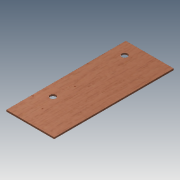
# Autodesk Inventor part: gabarito-contraponto
Saved by Autodesk Inventor 2017 (Build 210142000, 142)
## iProperties
Created: 2018-08-18
Part Number: gabarito-contraponto
Material: Wood (Oak)
Document SubType Name: Sheet Metal
Designer: Luiz Gustavo
Density: 0.76 g/cm^3
Sheet Metal Rule: Default_mm
Appearance: White Oak - Natural Medium Gloss
Author: Luiz Gustavo
Autodesk Inventor part; units mm, degrees
ref_plane "YZ Plane" through (0, 0, 0) normal (1, 0, 0) x (0, 1, 0)
ref_plane "XZ Plane" through (0, 0, 0) normal (0, 1, 0) x (-1, 0, 0)
ref_plane "XY Plane" through (0, 0, 0) normal (0, 0, 1) x (1, 0, 0)
sketch "Sketch1" plane through (0, 0, 0) normal (0, 0, 1) x (1, 0, 0)
  line L0 (-7.6357, 22.9943) -> (-8.4175, 23.9734) construction
  arc A0 (-7.6357, 22.9943) -> (-7.6357, 20.0058) centre (-4.4375, 21.5001) ccw construction
  line L1 (-8.4175, 19.0267) -> (-7.6357, 20.0058) construction
  arc A1 (-8.4175, 19.0267) -> (-6.9109, 17.5201) centre (-7.5798, 18.3578) ccw construction
  line L2 (-5.9318, 18.3019) -> (-6.9109, 17.5201) construction
  arc A2 (-5.9318, 18.3019) -> (-2.9433, 18.3019) centre (-4.4375, 21.5001) ccw construction
  line L3 (-1.9642, 17.5201) -> (-2.9433, 18.3019) construction
  arc A3 (-1.9642, 17.5201) -> (-0.4576, 19.0267) centre (-1.2953, 18.3578) ccw construction
  line L4 (-1.2394, 20.0058) -> (-0.4576, 19.0267) construction
  arc A4 (-1.2394, 20.0058) -> (-1.2394, 22.9943) centre (-4.4375, 21.5001) ccw construction
  line L5 (-0.4576, 23.9734) -> (-1.2394, 22.9943) construction
  arc A5 (-0.4576, 23.9734) -> (-1.9642, 25.48) centre (-1.2953, 24.6423) ccw construction
  line L6 (-2.9433, 24.6982) -> (-1.9642, 25.48) construction
  arc A6 (-2.9433, 24.6982) -> (-5.9318, 24.6982) centre (-4.4375, 21.5001) ccw construction
  line L7 (-6.9109, 25.48) -> (-5.9318, 24.6982) construction
  arc A7 (-6.9109, 25.48) -> (-8.4175, 23.9734) centre (-7.5798, 24.6423) ccw construction
  line L8 (-18.1375, 31.381) -> (-18.1375, 34.2) construction
  arc A8 (-18.1375, 31.381) -> (-17.7565, 31) centre (-17.7565, 31.381) ccw construction
  line L9 (-14.3175, 31) -> (-17.7565, 31) construction
  arc A9 (-14.3175, 31) -> (-13.9375, 31.38) centre (-14.3175, 31.38) ccw construction
  line L10 (-13.9375, 34.819) -> (-13.9375, 31.38) construction
  arc A10 (-13.9375, 34.819) -> (-14.3185, 35.2) centre (-14.3185, 34.819) ccw construction
  line L11 (-17.1375, 35.2) -> (-14.3185, 35.2) construction
  arc A11 (-17.1375, 35.2) -> (-18.1375, 34.2) centre (-17.1375, 34.2) ccw construction
  line L12 (9.2624, 11.6191) -> (9.2624, 8.8001) construction
  arc A12 (9.2624, 11.6191) -> (8.8814, 12.0001) centre (8.8814, 11.6191) ccw construction
  line L13 (5.4424, 12.0001) -> (8.8814, 12.0001) construction
  arc A13 (5.4424, 12.0001) -> (5.0624, 11.6201) centre (5.4424, 11.6201) ccw construction
  line L14 (5.0624, 8.1811) -> (5.0624, 11.6201) construction
  arc A14 (5.0624, 8.1811) -> (5.4434, 7.8001) centre (5.4434, 8.1811) ccw construction
  line L15 (8.2624, 7.8001) -> (5.4434, 7.8001) construction
  arc A15 (8.2624, 7.8001) -> (9.2624, 8.8001) centre (8.2624, 8.8001) ccw construction
  line L16 (-14.3185, 7.8001) -> (-17.1375, 7.8001) construction
  arc A16 (-14.3185, 7.8001) -> (-13.9375, 8.1811) centre (-14.3185, 8.1811) ccw construction
  line L17 (-13.9375, 11.6201) -> (-13.9375, 8.1811) construction
  arc A17 (-13.9375, 11.6201) -> (-14.3175, 12.0001) centre (-14.3175, 11.6201) ccw construction
  line L18 (-17.7565, 12.0001) -> (-14.3175, 12.0001) construction
  arc A18 (-17.7565, 12.0001) -> (-18.1375, 11.6191) centre (-17.7565, 11.6191) ccw construction
  line L19 (-18.1375, 8.8001) -> (-18.1375, 11.6191) construction
  arc A19 (-18.1375, 8.8001) -> (-17.1375, 7.8001) centre (-17.1375, 8.8001) ccw construction
  line L20 (8.8814, 31) -> (5.4424, 31) construction
  arc A20 (8.8814, 31) -> (9.2624, 31.381) centre (8.8814, 31.381) ccw construction
  line L21 (9.2624, 34.2) -> (9.2624, 31.381) construction
  arc A21 (9.2624, 34.2) -> (8.2624, 35.2) centre (8.2624, 34.2) ccw construction
  line L22 (5.4434, 35.2) -> (8.2624, 35.2) construction
  arc A22 (5.4434, 35.2) -> (5.0624, 34.819) centre (5.4434, 34.819) ccw construction
  line L23 (5.0624, 31.38) -> (5.0624, 34.819) construction
  arc A23 (5.0624, 31.38) -> (5.4424, 31) centre (5.4424, 31.38) ccw construction
  line L24 (0.0625, 34.2425) -> (3.295, 34.2425) construction
  arc A24 (-0.4375, 34.7425) -> (0.0625, 34.2425) centre (0.0625, 34.7425) ccw construction
  line L25 (-0.4375, 36) -> (-0.4375, 34.7425) construction
  arc A25 (0.0625, 36.5) -> (-0.4375, 36) centre (0.0625, 36) ccw construction
  line L26 (8.5624, 36.5) -> (0.0625, 36.5) construction
  arc A26 (10.5624, 34.5) -> (8.5624, 36.5) centre (8.5624, 34.5) ccw construction
  line L27 (10.5624, 26.0001) -> (10.5624, 34.5) construction
  arc A27 (10.0624, 25.5001) -> (10.5624, 26.0001) centre (10.0624, 26.0001) ccw construction
  line L28 (8.8049, 25.5001) -> (10.0624, 25.5001) construction
  arc A28 (8.3049, 26.0001) -> (8.8049, 25.5001) centre (8.8049, 26.0001) ccw construction
  line L29 (8.3049, 29.2326) -> (8.3049, 26.0001) construction
  arc A29 (8.3049, 29.2326) -> (7.8053, 29.75) centre (7.8053, 29.25) ccw construction
  line L30 (5.8227, 29.75) -> (7.8053, 29.75) construction
  arc A30 (5.8227, 29.75) -> (5.4691, 29.6036) centre (5.8227, 29.25) ccw construction
  line L31 (1.5436, 25.6781) -> (5.4691, 29.6036) construction
  arc A31 (1.5436, 25.6781) -> (1.3971, 25.3245) centre (1.8971, 25.3245) ccw construction
  line L32 (1.3971, 22.4501) -> (1.3971, 25.3245) construction
  line L33 (0.8871, 21.5001) -> (1.3971, 22.4501) construction
  line L34 (1.3971, 20.5501) -> (0.8871, 21.5001) construction
  line L35 (1.3971, 17.6756) -> (1.3971, 20.5501) construction
  arc A32 (1.3971, 17.6756) -> (1.5436, 17.3221) centre (1.8971, 17.6756) ccw construction
  line L36 (5.4691, 13.3965) -> (1.5436, 17.3221) construction
  arc A33 (5.4691, 13.3965) -> (5.8227, 13.2501) centre (5.8227, 13.7501) ccw construction
  line L37 (7.8053, 13.2501) -> (5.8227, 13.2501) construction
  arc A34 (7.8053, 13.2501) -> (8.3049, 13.7675) centre (7.8053, 13.7501) ccw construction
  line L38 (8.3049, 17.0001) -> (8.3049, 13.7675) construction
  arc A35 (8.8049, 17.5001) -> (8.3049, 17.0001) centre (8.8049, 17.0001) ccw construction
  line L39 (10.0624, 17.5001) -> (8.8049, 17.5001) construction
  arc A36 (10.5624, 17.0001) -> (10.0624, 17.5001) centre (10.0624, 17.0001) ccw construction
  line L40 (10.5624, 8.5001) -> (10.5624, 17.0001) construction
  arc A37 (8.5624, 6.5001) -> (10.5624, 8.5001) centre (8.5624, 8.5001) ccw construction
  line L41 (0.0625, 6.5001) -> (8.5624, 6.5001) construction
  arc A38 (-0.4375, 7.0001) -> (0.0625, 6.5001) centre (0.0625, 7.0001) ccw construction
  line L42 (-0.4375, 8.2576) -> (-0.4375, 7.0001) construction
  arc A39 (0.0625, 8.7576) -> (-0.4375, 8.2576) centre (0.0625, 8.2576) ccw construction
  line L43 (3.295, 8.7576) -> (0.0625, 8.7576) construction
  arc A40 (3.295, 8.7576) -> (3.8124, 9.2573) centre (3.3124, 9.2573) ccw construction
  line L44 (3.8124, 11.2399) -> (3.8124, 9.2573) construction
  arc A41 (3.8124, 11.2399) -> (3.666, 11.5934) centre (3.3124, 11.2399) ccw construction
  line L45 (-0.2595, 15.5189) -> (3.666, 11.5934) construction
  arc A42 (-0.2595, 15.5189) -> (-0.6131, 15.6654) centre (-0.6131, 15.1654) ccw construction
  line L46 (-3.55, 15.6654) -> (-0.6131, 15.6654) construction
  line L47 (-4.5, 16.1754) -> (-3.55, 15.6654) construction
  line L48 (-5.45, 15.6654) -> (-4.5, 16.1754) construction
  line L49 (-8.262, 15.6654) -> (-5.45, 15.6654) construction
  arc A43 (-8.262, 15.6654) -> (-8.6155, 15.5189) centre (-8.262, 15.1654) ccw construction
  line L50 (-12.5411, 11.5934) -> (-8.6155, 15.5189) construction
  arc A44 (-12.5411, 11.5934) -> (-12.6875, 11.2399) centre (-12.1875, 11.2399) ccw construction
  line L51 (-12.6875, 9.2573) -> (-12.6875, 11.2399) construction
  arc A45 (-12.6875, 9.2573) -> (-12.17, 8.7576) centre (-12.1875, 9.2573) ccw construction
  line L52 (-8.9375, 8.7576) -> (-12.17, 8.7576) construction
  arc A46 (-8.4375, 8.2576) -> (-8.9375, 8.7576) centre (-8.9375, 8.2576) ccw construction
  line L53 (-8.4375, 7.0001) -> (-8.4375, 8.2576) construction
  arc A47 (-8.9375, 6.5001) -> (-8.4375, 7.0001) centre (-8.9375, 7.0001) ccw construction
  line L54 (-17.4375, 6.5001) -> (-8.9375, 6.5001) construction
  arc A48 (-19.4375, 8.5001) -> (-17.4375, 6.5001) centre (-17.4375, 8.5001) ccw construction
  line L55 (-19.4375, 17.0001) -> (-19.4375, 8.5001) construction
  arc A49 (-18.9375, 17.5001) -> (-19.4375, 17.0001) centre (-18.9375, 17.0001) ccw construction
  line L56 (-17.68, 17.5001) -> (-18.9375, 17.5001) construction
  arc A50 (-17.18, 17.0001) -> (-17.68, 17.5001) centre (-17.68, 17.0001) ccw construction
  line L57 (-17.18, 13.7675) -> (-17.18, 17.0001) construction
  arc A51 (-17.18, 13.7675) -> (-16.6803, 13.2501) centre (-16.6803, 13.7501) ccw construction
  line L58 (-14.6977, 13.2501) -> (-16.6803, 13.2501) construction
  arc A52 (-14.6977, 13.2501) -> (-14.3442, 13.3965) centre (-14.6977, 13.7501) ccw construction
  line L59 (-10.4186, 17.3221) -> (-14.3442, 13.3965) construction
  arc A53 (-10.4186, 17.3221) -> (-10.2722, 17.6756) centre (-10.7722, 17.6756) ccw construction
  line L60 (-10.2722, 20.5501) -> (-10.2722, 17.6756) construction
  line L61 (-9.7622, 21.5001) -> (-10.2722, 20.5501) construction
  line L62 (-10.2722, 22.4501) -> (-9.7622, 21.5001) construction
  line L63 (-10.2722, 25.3245) -> (-10.2722, 22.4501) construction
  arc A54 (-10.2722, 25.3245) -> (-10.4186, 25.6781) centre (-10.7722, 25.3245) ccw construction
  line L64 (-14.3442, 29.6036) -> (-10.4186, 25.6781) construction
  arc A55 (-14.3442, 29.6036) -> (-14.6977, 29.75) centre (-14.6977, 29.25) ccw construction
  line L65 (-16.6803, 29.75) -> (-14.6977, 29.75) construction
  arc A56 (-16.6803, 29.75) -> (-17.18, 29.2326) centre (-16.6803, 29.25) ccw construction
  line L66 (-17.18, 26.0001) -> (-17.18, 29.2326) construction
  arc A57 (-17.68, 25.5001) -> (-17.18, 26.0001) centre (-17.68, 26.0001) ccw construction
  line L67 (-18.9375, 25.5001) -> (-17.68, 25.5001) construction
  arc A58 (-19.4375, 26.0001) -> (-18.9375, 25.5001) centre (-18.9375, 26.0001) ccw construction
  line L68 (-19.4375, 34.5) -> (-19.4375, 26.0001) construction
  arc A59 (-17.4375, 36.5) -> (-19.4375, 34.5) centre (-17.4375, 34.5) ccw construction
  line L69 (-8.9375, 36.5) -> (-17.4375, 36.5) construction
  arc A60 (-8.4375, 36) -> (-8.9375, 36.5) centre (-8.9375, 36) ccw construction
  line L70 (-8.4375, 34.7425) -> (-8.4375, 36) construction
  arc A61 (-8.9375, 34.2425) -> (-8.4375, 34.7425) centre (-8.9375, 34.7425) ccw construction
  line L71 (-12.17, 34.2425) -> (-8.9375, 34.2425) construction
  arc A62 (-12.17, 34.2425) -> (-12.6875, 33.7428) centre (-12.1875, 33.7428) ccw construction
  line L72 (-12.6875, 31.7602) -> (-12.6875, 33.7428) construction
  arc A63 (-12.6875, 31.7602) -> (-12.5411, 31.4067) centre (-12.1875, 31.7602) ccw construction
  line L73 (-8.6155, 27.4812) -> (-12.5411, 31.4067) construction
  arc A64 (-8.6155, 27.4812) -> (-8.262, 27.3347) centre (-8.262, 27.8347) ccw construction
  line L74 (-5.45, 27.3347) -> (-8.262, 27.3347) construction
  line L75 (-4.5, 26.8247) -> (-5.45, 27.3347) construction
  line L76 (-3.55, 27.3347) -> (-4.5, 26.8247) construction
  line L77 (-0.6131, 27.3347) -> (-3.55, 27.3347) construction
  arc A65 (-0.6131, 27.3347) -> (-0.2595, 27.4812) centre (-0.6131, 27.8347) ccw construction
  line L78 (3.666, 31.4067) -> (-0.2595, 27.4812) construction
  arc A66 (3.666, 31.4067) -> (3.8124, 31.7602) centre (3.3124, 31.7602) ccw construction
  line L79 (3.8124, 33.7428) -> (3.8124, 31.7602) construction
  arc A67 (3.8124, 33.7428) -> (3.295, 34.2425) centre (3.3124, 33.7428) ccw construction
  line L80 (-7.6357, 110.0057) -> (-8.4175, 109.0266) construction
  arc A68 (-8.4175, 109.0266) -> (-6.9109, 107.52) centre (-7.5798, 108.3577) ccw construction
  line L81 (-6.9109, 107.52) -> (-5.9318, 108.3018) construction
  arc A69 (-5.9318, 108.3018) -> (-2.9433, 108.3018) centre (-4.4375, 111.4999) ccw construction
  line L82 (-2.9433, 108.3018) -> (-1.9642, 107.52) construction
  arc A70 (-1.9642, 107.52) -> (-0.4576, 109.0266) centre (-1.2953, 108.3577) ccw construction
  line L83 (-0.4576, 109.0266) -> (-1.2394, 110.0057) construction
  arc A71 (-1.2394, 110.0057) -> (-1.2394, 112.9942) centre (-4.4375, 111.4999) ccw construction
  line L84 (-1.2394, 112.9942) -> (-0.4576, 113.9733) construction
  arc A72 (-0.4576, 113.9733) -> (-1.9642, 115.4799) centre (-1.2953, 114.6422) ccw construction
  line L85 (-1.9642, 115.4799) -> (-2.9433, 114.6981) construction
  arc A73 (-2.9433, 114.6981) -> (-5.9318, 114.6981) centre (-4.4375, 111.4999) ccw construction
  line L86 (-5.9318, 114.6981) -> (-6.9109, 115.4799) construction
  arc A74 (-6.9109, 115.4799) -> (-8.4175, 113.9733) centre (-7.5798, 114.6422) ccw construction
  line L87 (-8.4175, 113.9733) -> (-7.6357, 112.9942) construction
  arc A75 (-7.6357, 112.9942) -> (-7.6357, 110.0057) centre (-4.4375, 111.4999) ccw construction
  line L88 (-18.1375, 101.619) -> (-18.1375, 98.8) construction
  arc A76 (-18.1375, 98.8) -> (-17.1375, 97.8) centre (-17.1375, 98.8) ccw construction
  line L89 (-17.1375, 97.8) -> (-14.3185, 97.8) construction
  arc A77 (-14.3185, 97.8) -> (-13.9375, 98.181) centre (-14.3185, 98.181) ccw construction
  line L90 (-13.9375, 98.181) -> (-13.9375, 101.62) construction
  arc A78 (-13.9375, 101.62) -> (-14.3175, 102) centre (-14.3175, 101.62) ccw construction
  line L91 (-14.3175, 102) -> (-17.7565, 102) construction
  arc A79 (-17.7565, 102) -> (-18.1375, 101.619) centre (-17.7565, 101.619) ccw construction
  line L92 (9.2624, 121.3809) -> (9.2624, 124.1999) construction
  arc A80 (9.2624, 124.1999) -> (8.2624, 125.1999) centre (8.2624, 124.1999) ccw construction
  line L93 (8.2624, 125.1999) -> (5.4434, 125.1999) construction
  arc A81 (5.4434, 125.1999) -> (5.0624, 124.8189) centre (5.4434, 124.8189) ccw construction
  line L94 (5.0624, 124.8189) -> (5.0624, 121.3799) construction
  arc A82 (5.0624, 121.3799) -> (5.4424, 120.9999) centre (5.4424, 121.3799) ccw construction
  line L95 (5.4424, 120.9999) -> (8.8814, 120.9999) construction
  arc A83 (8.8814, 120.9999) -> (9.2624, 121.3809) centre (8.8814, 121.3809) ccw construction
  line L96 (-14.3185, 125.1999) -> (-17.1375, 125.1999) construction
  arc A84 (-17.1375, 125.1999) -> (-18.1375, 124.1999) centre (-17.1375, 124.1999) ccw construction
  line L97 (-18.1375, 124.1999) -> (-18.1375, 121.3809) construction
  arc A85 (-18.1375, 121.3809) -> (-17.7565, 120.9999) centre (-17.7565, 121.3809) ccw construction
  line L98 (-17.7565, 120.9999) -> (-14.3175, 120.9999) construction
  arc A86 (-14.3175, 120.9999) -> (-13.9375, 121.3799) centre (-14.3175, 121.3799) ccw construction
  line L99 (-13.9375, 121.3799) -> (-13.9375, 124.8189) construction
  arc A87 (-13.9375, 124.8189) -> (-14.3185, 125.1999) centre (-14.3185, 124.8189) ccw construction
  line L100 (8.8814, 102) -> (5.4424, 102) construction
  arc A88 (5.4424, 102) -> (5.0624, 101.62) centre (5.4424, 101.62) ccw construction
  line L101 (5.0624, 101.62) -> (5.0624, 98.181) construction
  arc A89 (5.0624, 98.181) -> (5.4434, 97.8) centre (5.4434, 98.181) ccw construction
  line L102 (5.4434, 97.8) -> (8.2624, 97.8) construction
  arc A90 (8.2624, 97.8) -> (9.2624, 98.8) centre (8.2624, 98.8) ccw construction
  line L103 (9.2624, 98.8) -> (9.2624, 101.619) construction
  arc A91 (9.2624, 101.619) -> (8.8814, 102) centre (8.8814, 101.619) ccw construction
  line L104 (0.0625, 98.7575) -> (3.295, 98.7575) construction
  arc A92 (3.295, 98.7575) -> (3.8124, 99.2572) centre (3.3124, 99.2572) ccw construction
  line L105 (3.8124, 99.2572) -> (3.8124, 101.2398) construction
  arc A93 (3.8124, 101.2398) -> (3.666, 101.5933) centre (3.3124, 101.2398) ccw construction
  line L106 (3.666, 101.5933) -> (-0.2595, 105.5188) construction
  arc A94 (-0.2595, 105.5188) -> (-0.6131, 105.6653) centre (-0.6131, 105.1653) ccw construction
  line L107 (-0.6131, 105.6653) -> (-3.55, 105.6653) construction
  line L108 (-3.55, 105.6653) -> (-4.5, 106.1753) construction
  line L109 (-4.5, 106.1753) -> (-5.45, 105.6653) construction
  line L110 (-5.45, 105.6653) -> (-8.262, 105.6653) construction
  arc A95 (-8.262, 105.6653) -> (-8.6155, 105.5188) centre (-8.262, 105.1653) ccw construction
  line L111 (-8.6155, 105.5188) -> (-12.5411, 101.5933) construction
  arc A96 (-12.5411, 101.5933) -> (-12.6875, 101.2398) centre (-12.1875, 101.2398) ccw construction
  line L112 (-12.6875, 101.2398) -> (-12.6875, 99.2572) construction
  arc A97 (-12.6875, 99.2572) -> (-12.17, 98.7575) centre (-12.1875, 99.2572) ccw construction
  line L113 (-12.17, 98.7575) -> (-8.9375, 98.7575) construction
  arc A98 (-8.4375, 98.2575) -> (-8.9375, 98.7575) centre (-8.9375, 98.2575) ccw construction
  line L114 (-8.4375, 98.2575) -> (-8.4375, 97) construction
  arc A99 (-8.9375, 96.5) -> (-8.4375, 97) centre (-8.9375, 97) ccw construction
  line L115 (-8.9375, 96.5) -> (-17.4375, 96.5) construction
  arc A100 (-19.4375, 98.5) -> (-17.4375, 96.5) centre (-17.4375, 98.5) ccw construction
  line L116 (-19.4375, 98.5) -> (-19.4375, 106.9999) construction
  arc A101 (-18.9375, 107.4999) -> (-19.4375, 106.9999) centre (-18.9375, 106.9999) ccw construction
  line L117 (-18.9375, 107.4999) -> (-17.68, 107.4999) construction
  arc A102 (-17.18, 106.9999) -> (-17.68, 107.4999) centre (-17.68, 106.9999) ccw construction
  line L118 (-17.18, 106.9999) -> (-17.18, 103.7674) construction
  arc A103 (-17.18, 103.7674) -> (-16.6803, 103.25) centre (-16.6803, 103.75) ccw construction
  line L119 (-16.6803, 103.25) -> (-14.6977, 103.25) construction
  arc A104 (-14.6977, 103.25) -> (-14.3442, 103.3964) centre (-14.6977, 103.75) ccw construction
  line L120 (-14.3442, 103.3964) -> (-10.4186, 107.3219) construction
  arc A105 (-10.4186, 107.3219) -> (-10.2722, 107.6755) centre (-10.7722, 107.6755) ccw construction
  line L121 (-10.2722, 107.6755) -> (-10.2722, 110.5499) construction
  line L122 (-10.2722, 110.5499) -> (-9.7622, 111.4999) construction
  line L123 (-9.7622, 111.4999) -> (-10.2722, 112.4499) construction
  line L124 (-10.2722, 112.4499) -> (-10.2722, 115.3244) construction
  arc A106 (-10.2722, 115.3244) -> (-10.4186, 115.6779) centre (-10.7722, 115.3244) ccw construction
  line L125 (-10.4186, 115.6779) -> (-14.3442, 119.6035) construction
  arc A107 (-14.3442, 119.6035) -> (-14.6977, 119.7499) centre (-14.6977, 119.2499) ccw construction
  line L126 (-14.6977, 119.7499) -> (-16.6803, 119.7499) construction
  arc A108 (-16.6803, 119.7499) -> (-17.18, 119.2325) centre (-16.6803, 119.2499) ccw construction
  line L127 (-17.18, 119.2325) -> (-17.18, 115.9999) construction
  arc A109 (-17.68, 115.4999) -> (-17.18, 115.9999) centre (-17.68, 115.9999) ccw construction
  line L128 (-17.68, 115.4999) -> (-18.9375, 115.4999) construction
  arc A110 (-19.4375, 115.9999) -> (-18.9375, 115.4999) centre (-18.9375, 115.9999) ccw construction
  line L129 (-19.4375, 115.9999) -> (-19.4375, 124.4999) construction
  arc A111 (-17.4375, 126.4999) -> (-19.4375, 124.4999) centre (-17.4375, 124.4999) ccw construction
  line L130 (-17.4375, 126.4999) -> (-8.9375, 126.4999) construction
  arc A112 (-8.4375, 125.9999) -> (-8.9375, 126.4999) centre (-8.9375, 125.9999) ccw construction
  line L131 (-8.4375, 125.9999) -> (-8.4375, 124.7424) construction
  arc A113 (-8.9375, 124.2424) -> (-8.4375, 124.7424) centre (-8.9375, 124.7424) ccw construction
  line L132 (-8.9375, 124.2424) -> (-12.17, 124.2424) construction
  arc A114 (-12.17, 124.2424) -> (-12.6875, 123.7427) centre (-12.1875, 123.7427) ccw construction
  line L133 (-12.6875, 123.7427) -> (-12.6875, 121.7601) construction
  arc A115 (-12.6875, 121.7601) -> (-12.5411, 121.4066) centre (-12.1875, 121.7601) ccw construction
  line L134 (-12.5411, 121.4066) -> (-8.6155, 117.4811) construction
  arc A116 (-8.6155, 117.4811) -> (-8.262, 117.3346) centre (-8.262, 117.8346) ccw construction
  line L135 (-8.262, 117.3346) -> (-5.45, 117.3346) construction
  line L136 (-5.45, 117.3346) -> (-4.5, 116.8246) construction
  line L137 (-4.5, 116.8246) -> (-3.55, 117.3346) construction
  line L138 (-3.55, 117.3346) -> (-0.6131, 117.3346) construction
  arc A117 (-0.6131, 117.3346) -> (-0.2595, 117.4811) centre (-0.6131, 117.8346) ccw construction
  line L139 (-0.2595, 117.4811) -> (3.666, 121.4066) construction
  arc A118 (3.666, 121.4066) -> (3.8124, 121.7601) centre (3.3124, 121.7601) ccw construction
  line L140 (3.8124, 121.7601) -> (3.8124, 123.7427) construction
  arc A119 (3.8124, 123.7427) -> (3.295, 124.2424) centre (3.3124, 123.7427) ccw construction
  line L141 (3.295, 124.2424) -> (0.0625, 124.2424) construction
  arc A120 (-0.4375, 124.7424) -> (0.0625, 124.2424) centre (0.0625, 124.7424) ccw construction
  line L142 (-0.4375, 124.7424) -> (-0.4375, 125.9999) construction
  arc A121 (0.0625, 126.4999) -> (-0.4375, 125.9999) centre (0.0625, 125.9999) ccw construction
  line L143 (0.0625, 126.4999) -> (8.5624, 126.4999) construction
  arc A122 (10.5624, 124.4999) -> (8.5624, 126.4999) centre (8.5624, 124.4999) ccw construction
  line L144 (10.5624, 124.4999) -> (10.5624, 115.9999) construction
  arc A123 (10.0624, 115.4999) -> (10.5624, 115.9999) centre (10.0624, 115.9999) ccw construction
  line L145 (10.0624, 115.4999) -> (8.8049, 115.4999) construction
  arc A124 (8.3049, 115.9999) -> (8.8049, 115.4999) centre (8.8049, 115.9999) ccw construction
  line L146 (8.3049, 115.9999) -> (8.3049, 119.2325) construction
  arc A125 (8.3049, 119.2325) -> (7.8053, 119.7499) centre (7.8053, 119.2499) ccw construction
  line L147 (7.8053, 119.7499) -> (5.8227, 119.7499) construction
  arc A126 (5.8227, 119.7499) -> (5.4691, 119.6035) centre (5.8227, 119.2499) ccw construction
  line L148 (5.4691, 119.6035) -> (1.5436, 115.6779) construction
  arc A127 (1.5436, 115.6779) -> (1.3971, 115.3244) centre (1.8971, 115.3244) ccw construction
  line L149 (1.3971, 115.3244) -> (1.3971, 112.4499) construction
  line L150 (1.3971, 112.4499) -> (0.8871, 111.4999) construction
  line L151 (0.8871, 111.4999) -> (1.3971, 110.5499) construction
  line L152 (1.3971, 110.5499) -> (1.3971, 107.6755) construction
  arc A128 (1.3971, 107.6755) -> (1.5436, 107.3219) centre (1.8971, 107.6755) ccw construction
  line L153 (1.5436, 107.3219) -> (5.4691, 103.3964) construction
  arc A129 (5.4691, 103.3964) -> (5.8227, 103.25) centre (5.8227, 103.75) ccw construction
  line L154 (5.8227, 103.25) -> (7.8053, 103.25) construction
  arc A130 (7.8053, 103.25) -> (8.3049, 103.7674) centre (7.8053, 103.75) ccw construction
  line L155 (8.3049, 103.7674) -> (8.3049, 106.9999) construction
  arc A131 (8.8049, 107.4999) -> (8.3049, 106.9999) centre (8.8049, 106.9999) ccw construction
  line L156 (8.8049, 107.4999) -> (10.0624, 107.4999) construction
  arc A132 (10.5624, 106.9999) -> (10.0624, 107.4999) centre (10.0624, 106.9999) ccw construction
  line L157 (10.5624, 106.9999) -> (10.5624, 98.5) construction
  arc A133 (8.5624, 96.5) -> (10.5624, 98.5) centre (8.5624, 98.5) ccw construction
  line L158 (8.5624, 96.5) -> (0.0625, 96.5) construction
  arc A134 (-0.4375, 97) -> (0.0625, 96.5) centre (0.0625, 97) ccw construction
  line L159 (-0.4375, 97) -> (-0.4375, 98.2575) construction
  arc A135 (0.0625, 98.7575) -> (-0.4375, 98.2575) centre (0.0625, 98.2575) ccw construction
  line L160 (0.125, 128.0008) -> (20.9999, 128.0008) construction
  ellipse E0 centre (-17.4375, -22.0067) end of major axis (-15.4375, -22.0067) minor radius 0.0008 (-19.4375, -22.0067) -> (-17.4375, -22.0075) ccw construction
  line L161 (40.5624, -22.0067) -> (40.5624, 127.9901)
  line L162 (-19.4375, -22.0067) -> (40.5624, -22.0067)
  line L163 (40.5624, -22.0067) -> (40.5624, 127.9901)
  line L164 (40.5624, 127.9901) -> (-19.4375, 127.9901)
  line L165 (-19.4375, 127.9901) -> (-19.4375, -22.0067)
  circle A136 centre (-4.4375, 111.4999) radius 3.75
  circle A137 centre (-4.4375, 21.5001) radius 3.75
  point P0 (0, 0)
  dimension "d0" = 59.9999
  dimension "d1" = 7.5
  measures "d0" distance of L161.end L164.end
  measures "d1" diameter of A136
extrude "Plate1" add sketch "Sketch1" along normal blind 2
equation "\"BendRadius\" = Thickness"
equation "\"BendReliefWidth\" = Thickness"
equation "\"BendReliefDepth\" = 0.5 * Thickness"
equation "\"CornerReliefSize\" = 4 * Thickness"
equation "\"MinimumRemnant\" = 2 * Thickness"
equation "\"TransitionRadius\" = BendRadius"
equation "\"JacobiRadiusSize\" = BendRadius"
equation "\"GapSize\" = Thickness"
equation "\"d2\" = BendRadius"
equation "\"Thickness\" = 2"
body "Solid1"
